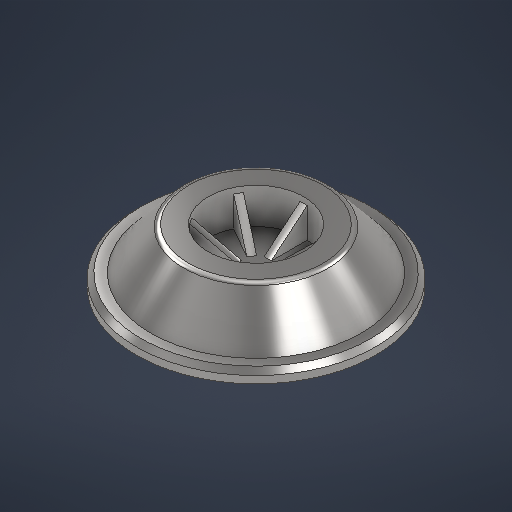
# Autodesk Inventor part: ensayo11
Saved by Autodesk Inventor 2026.2 (Build 302298000, 298)
## iProperties
Created: 2025-12-23
Part Number: ensayo11
Material: Acero inoxidable
Document SubType Name: Modeling
Designer: vicho
Mass: 6174.44 g
Surface Area: 865.841 cm^2
Volume: 771.805 cm^3
Density: 8 g/cm^3
Appearance: Semipulido
Author: vicho
Autodesk Inventor part; units mm, degrees
note: some values were not read from the file. Chosen so that the rebuilt part matches the saved one: direction of "Repujado1".
ref_plane "YZ Plane" through (0, 0, 0) normal (1, 0, 0) x (0, 1, 0)
ref_plane "XY Plane" through (0, 0, 0) normal (0, 0, 1) x (1, 0, 0)
sketch "Boceto1" plane through (0, 0, 0) normal (0, 0, 1) x (1, 0, 0)
  line L0 (0, 50) -> (0, -50) construction
  line L1 (75, 0) -> (-75, 0) construction
  line L2 (-100, 0) -> (-100, 10)
  line L3 (-100, 10) -> (-88, 10)
  line L4 (-88, 10) -> (-58.7804, 45)
  line L5 (-58.7804, 45) -> (-40, 45)
  line L6 (-40, 45) -> (-40, 40.173)
  line L7 (-40, 40.173) -> (-10, 15)
  line L8 (-10, 15) -> (0, 15)
  line L9 (-100, 0) -> (0, 0)
  line L10 (0, 15) -> (-75.8865, 15) construction
  line L11 (0, 15) -> (0, 0)
  dimension "d0" = 150
  dimension "d1" = 100
  dimension "d4" = 10
  dimension "d5" = 15
  dimension "d6" = 10
  dimension "d7" = 12
  dimension "d8" = 45
  dimension "d9" = 40
  dimension "d10" = 40
  dimension "d11" = 100
  dimension "d14" = 39.857
  dimension "d15" = 0
  dimension "d16" = 75.8865
  constraints: 24 end point, 3 perpendicular, 3 point on line, 2 parallel, 2 symmetric about line, 2 vertical, 1 horizontal, 1 midpoint
  measures "d0" distance of L1.start L1.end
  measures "d1" distance of L0.end L0.start
  measures "d4" distance from line of L0 L7.end
  measures "d5" distance between parallel lines of L1 L8
  measures "d6" distance from line of L9 L2.end
  measures "d7" distance of L3.end L2.end
  measures "d8" distance between parallel lines of L1 L5
  measures "d9" distance between parallel lines of L0 L6
  measures "d10" angle of L10 L7
  measures "d11" distance between parallel lines of L0 L2
  measures "d14" angle of L4 L0
  measures "d15" distance from line of L9.end L0
  measures "d16" distance from line of L10.end L0
revolve "Revolución1" add sketch "Boceto1" angle 360 about axis through (0, 50, 0) along (0, -1, 0)
fillet "Empalme1" radius 5 1 edges at (58.7804, 45, 0)
chamfer "Chaflán1" distance 4 angle 45 1 edges at (100, 10, 0)
ref_plane "Plano de trabajo1" through (0, 45, 0) normal (0, 1, 0) x (-1, 0, 0)
sketch "Boceto2" plane through (0, 45, 0) normal (0, 1, 0) x (-1, 0, 0)
  line L0 (0, 63.6119) -> (0, -62.4959) construction
  line L1 (-64.3931, 0) -> (90.5075, 0) construction
  circle A0 centre (0, 0) radius 10 projected
  circle A1 centre (0, 0) radius 40
  line L2 (-3, -39.8873) -> (-3, -9.8873)
  line L3 (-3, -9.8873) -> (3, -9.8873)
  line L4 (3, -9.8873) -> (3, -39.8873)
  line L5 (10.0627, -2.3456) -> (36.0435, -17.3456)
  line L6 (33.0435, -22.5417) -> (7.0627, -7.5417)
  line L7 (7.0627, -7.5417) -> (10.0627, -2.3456)
  circle A2 centre (0, 0) radius 40
  line L8 (7.0627, 7.5417) -> (33.0435, 22.5417)
  line L9 (36.0435, 17.3456) -> (10.0627, 2.3456)
  line L10 (10.0627, 2.3456) -> (7.0627, 7.5417)
  circle A3 centre (0, 0) radius 40
  line L11 (-3, 9.8873) -> (-3, 39.8873)
  line L12 (3, 39.8873) -> (3, 9.8873)
  line L13 (3, 9.8873) -> (-3, 9.8873)
  circle A4 centre (0, 0) radius 40
  line L14 (-10.0627, 2.3456) -> (-36.0435, 17.3456)
  line L15 (-33.0435, 22.5417) -> (-7.0627, 7.5417)
  line L16 (-7.0627, 7.5417) -> (-10.0627, 2.3456)
  circle A5 centre (0, 0) radius 40
  line L17 (-7.0627, -7.5417) -> (-33.0435, -22.5417)
  line L18 (-36.0435, -17.3456) -> (-10.0627, -2.3456)
  line L19 (-10.0627, -2.3456) -> (-7.0627, -7.5417)
  circle A6 centre (0, 0) radius 40
  point P0 (-9.3111, -3.6474)
  point P1 (-9.3111, 3.6474)
  point P2 (-7.8143, -6.24)
  point P3 (-1.4968, -9.8873)
  point P4 (7.8143, -6.24)
  point P5 (1.4968, -9.8873)
  point P6 (9.3111, 3.6474)
  point P7 (9.3111, -3.6474)
  point P8 (-7.8143, 6.24)
  point P9 (-1.4968, 9.8873)
  point P10 (1.4968, 9.8873)
  point P11 (7.8143, 6.24)
  dimension "d23" = 80
  dimension "d24" = 6
  dimension "d25" = 30
  dimension "d28" = 360
  constraints: 40 end point, 12 point on circle, 6 centre point, 2 horizontal, 2 perpendicular, 2 vertical, 1 coincident, 1 parallel, 56 other
  measures "d23" diameter of A1
  measures "d24" distance between parallel lines of L4 L2
  measures "d25" distance from line of L2.start L3
extrude "Extrusión1" cut sketch "Boceto2" against normal blind 30 contours A0 L10 L9 A1 L5 L7 | A0 L13 L12 A1 L8 L10 | L7 L6 A1 L4 L3 A0 | A0 L16 L15 A1 L11 L13 | L3 L2 A1 L17 L19 A0 | A0 L19 L18 A1 L14 L16
sketch "Boceto3" plane through (0, 0, 0) normal (0, -1, 0) x (1, 0, 0)
  line L0 (0.5512, 0) -> (66.3296, 0) construction
  line L1 (66.3296, 0) -> (66.3296, -47.772) construction
  line L2 (66.3296, -47.772) -> (0.5512, -47.772) construction
  line L3 (0.5512, -47.772) -> (0.5512, 0) construction
  line L4 (0.454, -15.6686) -> (5.5107, -0.6686)
  line L5 (5.5107, -0.6686) -> (7.9661, -0.6686)
  line L6 (7.9661, -0.6686) -> (13.0229, -15.6686)
  line L7 (13.0229, -15.6686) -> (10.9199, -15.6686)
  line L8 (10.9199, -15.6686) -> (9.5585, -11.4749)
  line L9 (9.5585, -11.4749) -> (3.8332, -11.4749)
  line L10 (3.8332, -11.4749) -> (2.4718, -15.6686)
  line L11 (2.4718, -15.6686) -> (0.454, -15.6686)
  line L12 (9.0115, -9.7731) -> (6.6898, -2.7107)
  line L13 (6.6898, -2.7107) -> (4.3802, -9.7731)
  line L14 (4.3802, -9.7731) -> (9.0115, -9.7731)
  line L15 (23.0512, -15.6686) -> (21.1549, -15.6686)
  line L16 (21.1549, -15.6686) -> (21.1549, -14.4287)
  spline S0 degree 2 poles (21.1549, -14.4287) (20.2797, -15.1945) (18.7117, -15.9846) (17.7392, -15.9846) knots 0 0 0 1 2 2 2
  spline S1 degree 2 poles (17.7392, -15.9846) (17.0099, -15.9846) (15.7092, -15.4984) (15.2352, -14.9757) knots 0 0 0 1 2 2 2
  spline S2 degree 2 poles (15.2352, -14.9757) (14.7489, -14.453) (14.2141, -12.8606) (14.2141, -11.718) knots 0 0 0 1 2 2 2
  line L17 (14.2141, -11.718) -> (14.2141, -4.4125)
  line L18 (14.2141, -4.4125) -> (16.1104, -4.4125)
  line L19 (16.1104, -4.4125) -> (16.1104, -10.8306)
  spline S3 degree 2 poles (16.1104, -10.8306) (16.1104, -11.7301) (16.2441, -12.9092) (16.475, -13.3468) knots 0 0 0 1 2 2 2
  spline S4 degree 2 poles (16.475, -13.3468) (16.706, -13.7844) (17.4961, -14.1856) (18.2376, -14.1856) knots 0 0 0 1 2 2 2
  spline S5 degree 2 poles (18.2376, -14.1856) (18.9305, -14.1856) (20.4985, -13.3955) (21.1549, -12.8241) knots 0 0 0 1 2 2 2
  line L20 (21.1549, -12.8241) -> (21.1549, -4.4125)
  line L21 (21.1549, -4.4125) -> (23.0512, -4.4125)
  line L22 (23.0512, -4.4125) -> (23.0512, -15.6686)
  spline S6 degree 2 poles (29.2019, -15.8874) (27.6582, -15.8874) (25.9199, -14.1248) (25.9199, -12.2164) knots 0 0 0 1 2 2 2
  line L23 (25.9199, -12.2164) -> (25.9199, -5.9806)
  line L24 (25.9199, -5.9806) -> (24.6436, -5.9806)
  line L25 (24.6436, -5.9806) -> (24.6436, -4.4125)
  line L26 (24.6436, -4.4125) -> (25.9199, -4.4125)
  line L27 (25.9199, -4.4125) -> (25.9199, -1.1791)
  line L28 (25.9199, -1.1791) -> (27.8162, -1.1791)
  line L29 (27.8162, -1.1791) -> (27.8162, -4.4125)
  line L30 (27.8162, -4.4125) -> (31.3049, -4.4125)
  line L31 (31.3049, -4.4125) -> (31.3049, -5.9806)
  line L32 (31.3049, -5.9806) -> (27.8162, -5.9806)
  line L33 (27.8162, -5.9806) -> (27.8162, -11.3412)
  spline S7 degree 2 poles (27.8162, -11.3412) (27.8162, -12.1921) (27.877, -13.128) (28.0836, -13.5292) knots 0 0 0 1 2 2 2
  spline S8 degree 2 poles (28.0836, -13.5292) (28.2538, -13.8817) (29.0196, -14.2342) (29.676, -14.2342) knots 0 0 0 1 2 2 2
  spline S9 degree 2 poles (29.676, -14.2342) (30.1379, -14.2342) (31.001, -13.9546) (31.1955, -13.8695) knots 0 0 0 1 2 2 2
  line L34 (31.1955, -13.8695) -> (31.3049, -13.8695)
  line L35 (31.3049, -13.8695) -> (31.3049, -15.5713)
  spline S10 degree 2 poles (31.3049, -15.5713) (30.77, -15.7172) (29.676, -15.8874) (29.2019, -15.8874) knots 0 0 0 1 2 2 2
  spline S11 degree 2 poles (41.9532, -10.0405) (41.9532, -12.8849) (39.2182, -15.9846) (36.9329, -15.9846) knots 0 0 0 1 2 2 2
  spline S12 degree 2 poles (36.9329, -15.9846) (34.5869, -15.9846) (31.9005, -12.7877) (31.9005, -10.0405) knots 0 0 0 1 2 2 2
  spline S13 degree 2 poles (31.9005, -10.0405) (31.9005, -7.2204) (34.672, -4.0964) (36.9329, -4.0964) knots 0 0 0 1 2 2 2
  spline S14 degree 2 poles (36.9329, -4.0964) (39.2182, -4.0964) (41.9532, -7.2083) (41.9532, -10.0405) knots 0 0 0 1 2 2 2
  spline S15 degree 2 poles (39.9961, -10.0405) (39.9961, -7.8525) (38.4037, -5.7253) (36.9329, -5.7253) knots 0 0 0 1 2 2 2
  spline S16 degree 2 poles (36.9329, -5.7253) (35.4621, -5.7253) (33.8575, -7.8525) (33.8575, -10.0405) knots 0 0 0 1 2 2 2
  spline S17 degree 2 poles (33.8575, -10.0405) (33.8575, -12.1677) (35.4621, -14.3558) (36.9329, -14.3558) knots 0 0 0 1 2 2 2
  spline S18 degree 2 poles (36.9329, -14.3558) (38.3916, -14.3558) (39.9961, -12.2042) (39.9961, -10.0405) knots 0 0 0 1 2 2 2
  line L36 (52.5528, -15.6686) -> (50.6566, -15.6686)
  line L37 (50.6566, -15.6686) -> (50.6566, -14.5259)
  spline S19 degree 2 poles (50.6566, -14.5259) (50.219, -14.8906) (49.5747, -15.3768) (49.1371, -15.5835) knots 0 0 0 1 2 2 2
  spline S20 degree 2 poles (49.1371, -15.5835) (48.736, -15.778) (47.8729, -15.9846) (47.3016, -15.9846) knots 0 0 0 1 2 2 2
  spline S21 degree 2 poles (47.3016, -15.9846) (46.3778, -15.9846) (44.8219, -15.2188) (44.2749, -14.4773) knots 0 0 0 1 2 2 2
  spline S22 degree 2 poles (44.2749, -14.4773) (43.7279, -13.7358) (43.1201, -11.5478) (43.1201, -10.1256) knots 0 0 0 1 2 2 2
  spline S23 degree 2 poles (43.1201, -10.1256) (43.1201, -8.6426) (43.8859, -6.4789) (44.5545, -5.6645) knots 0 0 0 1 2 2 2
  spline S24 degree 2 poles (44.5545, -5.6645) (45.1744, -4.9352) (46.9126, -4.0964) (47.8729, -4.0964) knots 0 0 0 1 2 2 2
  spline S25 degree 2 poles (47.8729, -4.0964) (48.7117, -4.0964) (49.9637, -4.4733) (50.6566, -4.8622) knots 0 0 0 1 2 2 2
  line L38 (50.6566, -4.8622) -> (50.6566, 0)
  line L39 (50.6566, 0) -> (52.5528, 0)
  line L40 (52.5528, 0) -> (52.5528, -15.6686)
  line L41 (50.6566, -12.9335) -> (50.6566, -6.4303)
  spline S26 degree 2 poles (50.6566, -6.4303) (49.9515, -6.09) (48.8332, -5.8347) (48.189, -5.8347) knots 0 0 0 1 2 2 2
  spline S27 degree 2 poles (48.189, -5.8347) (46.7303, -5.8347) (45.0771, -8.0227) (45.0771, -10.0891) knots 0 0 0 1 2 2 2
  spline S28 degree 2 poles (45.0771, -10.0891) (45.0771, -12.0827) (46.3413, -14.1856) (47.7392, -14.1856) knots 0 0 0 1 2 2 2
  spline S29 degree 2 poles (47.7392, -14.1856) (48.4807, -14.1856) (49.988, -13.5049) (50.6566, -12.9335) knots 0 0 0 1 2 2 2
  spline S30 degree 2 poles (60.1865, -15.9238) (57.488, -15.9238) (54.522, -12.8971) (54.522, -10.1013) knots 0 0 0 1 2 2 2
  spline S31 degree 2 poles (54.522, -10.1013) (54.522, -7.3541) (57.4029, -4.0964) (59.7246, -4.0964) knots 0 0 0 1 2 2 2
  spline S32 degree 2 poles (59.7246, -4.0964) (60.77, -4.0964) (62.3867, -4.7042) (62.9823, -5.3485) knots 0 0 0 1 2 2 2
  spline S33 degree 2 poles (62.9823, -5.3485) (63.5901, -5.9927) (64.2344, -7.8525) (64.2344, -9.2018) knots 0 0 0 1 2 2 2
  line L42 (64.2344, -9.2018) -> (64.2344, -10.235)
  line L43 (64.2344, -10.235) -> (56.4426, -10.235)
  spline S34 degree 2 poles (56.4426, -10.235) (56.4426, -12.1921) (58.4118, -14.2707) (60.1622, -14.2707) knots 0 0 0 1 2 2 2
  spline S35 degree 2 poles (60.1622, -14.2707) (60.7822, -14.2707) (61.9856, -13.9911) (62.4718, -13.7723) knots 0 0 0 1 2 2 2
  spline S36 degree 2 poles (62.4718, -13.7723) (62.9823, -13.5292) (63.6874, -13.1037) (63.9183, -12.9092) knots 0 0 0 1 2 2 2
  line L44 (63.9183, -12.9092) -> (64.0277, -12.9092)
  line L45 (64.0277, -12.9092) -> (64.0277, -14.9757)
  spline S37 degree 2 poles (64.0277, -14.9757) (63.6995, -15.1094) (62.7028, -15.4984) (62.3138, -15.6078) knots 0 0 0 1 2 2 2
  spline S38 degree 2 poles (62.3138, -15.6078) (61.7668, -15.7658) (60.8673, -15.9238) (60.1865, -15.9238) knots 0 0 0 1 2 2 2
  spline S39 degree 2 poles (62.3867, -8.7885) (62.3624, -8.0227) (62.0464, -6.9044) (61.7425, -6.5276) knots 0 0 0 1 2 2 2
  spline S40 degree 2 poles (61.7425, -6.5276) (61.4143, -6.1021) (60.381, -5.6524) (59.6152, -5.6524) knots 0 0 0 1 2 2 2
  spline S41 degree 2 poles (59.6152, -5.6524) (58.8616, -5.6524) (57.8041, -6.1021) (57.3665, -6.5397) knots 0 0 0 1 2 2 2
  spline S42 degree 2 poles (57.3665, -6.5397) (56.941, -6.9895) (56.5034, -8.0713) (56.4426, -8.7885) knots 0 0 0 1 2 2 2
  line L46 (56.4426, -8.7885) -> (62.3867, -8.7885)
  spline S43 degree 2 poles (69.1938, -15.936) (68.0634, -15.936) (66.1063, -15.3282) (65.4621, -14.9878) knots 0 0 0 1 2 2 2
  line L47 (65.4621, -14.9878) -> (65.4621, -12.8606)
  line L48 (65.4621, -12.8606) -> (65.5593, -12.8606)
  spline S44 degree 2 poles (65.5593, -12.8606) (65.8024, -13.0551) (66.4588, -13.517) (67.0058, -13.7723) knots 0 0 0 1 2 2 2
  spline S45 degree 2 poles (67.0058, -13.7723) (67.4799, -14.0032) (68.6468, -14.3436) (69.2668, -14.3436) knots 0 0 0 1 2 2 2
  spline S46 degree 2 poles (69.2668, -14.3436) (69.7165, -14.3436) (70.7498, -14.137) (70.9929, -13.9668) knots 0 0 0 1 2 2 2
  spline S47 degree 2 poles (70.9929, -13.9668) (71.3454, -13.7358) (71.6614, -13.2131) (71.6614, -12.6783) knots 0 0 0 1 2 2 2
  spline S48 degree 2 poles (71.6614, -12.6783) (71.6614, -12.0097) (70.9321, -11.3169) (69.9961, -11.0859) knots 0 0 0 1 2 2 2
  spline S49 degree 2 poles (69.9961, -11.0859) (69.6314, -11.0008) (68.4645, -10.7577) (67.9661, -10.624) knots 0 0 0 1 2 2 2
  spline S50 degree 2 poles (67.9661, -10.624) (66.6776, -10.2472) (65.5107, -8.6912) (65.5107, -7.5851) knots 0 0 0 1 2 2 2
  spline S51 degree 2 poles (65.5107, -7.5851) (65.5107, -6.0535) (67.8081, -4.1451) (69.7044, -4.1451) knots 0 0 0 1 2 2 2
  spline S52 degree 2 poles (69.7044, -4.1451) (70.6404, -4.1451) (72.5366, -4.607) (73.1809, -4.9595) knots 0 0 0 1 2 2 2
  line L49 (73.1809, -4.9595) -> (73.1809, -6.9895)
  line L50 (73.1809, -6.9895) -> (73.0836, -6.9895)
  spline S53 degree 2 poles (73.0836, -6.9895) (72.3543, -6.406) (70.5796, -5.7374) (69.6679, -5.7374) knots 0 0 0 1 2 2 2
  spline S54 degree 2 poles (69.6679, -5.7374) (68.7319, -5.7374) (67.4434, -6.5276) (67.4434, -7.3177) knots 0 0 0 1 2 2 2
  spline S55 degree 2 poles (67.4434, -7.3177) (67.4434, -8.0348) (68.2092, -8.7277) (69.0601, -8.9465) knots 0 0 0 1 2 2 2
  spline S56 degree 2 poles (69.0601, -8.9465) (69.4734, -9.0559) (70.5188, -9.2747) (71.0901, -9.4084) knots 0 0 0 1 2 2 2
  spline S57 degree 2 poles (71.0901, -9.4084) (72.33, -9.7245) (73.5942, -11.171) (73.5942, -12.423) knots 0 0 0 1 2 2 2
  spline S58 degree 2 poles (73.5942, -12.423) (73.5942, -13.1524) (73.0229, -14.4408) (72.4637, -14.9149) knots 0 0 0 1 2 2 2
  spline S59 degree 2 poles (72.4637, -14.9149) (71.8681, -15.4133) (70.3486, -15.936) (69.1938, -15.936) knots 0 0 0 1 2 2 2
  line L51 (84.6801, -15.6686) -> (82.1882, -15.6686)
  line L52 (82.1882, -15.6686) -> (78.0066, -10.235)
  line L53 (78.0066, -10.235) -> (77.253, -10.9643)
  line L54 (77.253, -10.9643) -> (77.253, -15.6686)
  line L55 (77.253, -15.6686) -> (75.3567, -15.6686)
  line L56 (75.3567, -15.6686) -> (75.3567, 0)
  line L57 (75.3567, 0) -> (77.253, 0)
  line L58 (77.253, 0) -> (77.253, -9.1653)
  line L59 (77.253, -9.1653) -> (81.7019, -4.4125)
  line L60 (81.7019, -4.4125) -> (84.0601, -4.4125)
  line L61 (84.0601, -4.4125) -> (79.441, -9.1167)
  line L62 (79.441, -9.1167) -> (84.6801, -15.6686)
  line L63 (7.2976, -40.3657) -> (1.4872, -40.3657)
  line L64 (1.4872, -40.3657) -> (1.4872, -38.8341)
  line L65 (1.4872, -38.8341) -> (3.3956, -38.8341)
  line L66 (3.3956, -38.8341) -> (3.3956, -26.8973)
  line L67 (3.3956, -26.8973) -> (1.4872, -26.8973)
  line L68 (1.4872, -26.8973) -> (1.4872, -25.3657)
  line L69 (1.4872, -25.3657) -> (7.2976, -25.3657)
  line L70 (7.2976, -25.3657) -> (7.2976, -26.8973)
  line L71 (7.2976, -26.8973) -> (5.3891, -26.8973)
  line L72 (5.3891, -26.8973) -> (5.3891, -38.8341)
  line L73 (5.3891, -38.8341) -> (7.2976, -38.8341)
  line L74 (7.2976, -38.8341) -> (7.2976, -40.3657)
  line L75 (18.4564, -40.3657) -> (16.5601, -40.3657)
  line L76 (16.5601, -40.3657) -> (16.5601, -33.9475)
  spline S60 degree 2 poles (16.5601, -33.9475) (16.5601, -33.1696) (16.4143, -31.8324) (16.1955, -31.4313) knots 0 0 0 1 2 2 2
  spline S61 degree 2 poles (16.1955, -31.4313) (15.9645, -31.0059) (15.1379, -30.5926) (14.4329, -30.5926) knots 0 0 0 1 2 2 2
  spline S62 degree 2 poles (14.4329, -30.5926) (13.7279, -30.5926) (12.2327, -31.3462) (11.5156, -31.954) knots 0 0 0 1 2 2 2
  line L77 (11.5156, -31.954) -> (11.5156, -40.3657)
  line L78 (11.5156, -40.3657) -> (9.6193, -40.3657)
  line L79 (9.6193, -40.3657) -> (9.6193, -29.1096)
  line L80 (9.6193, -29.1096) -> (11.5156, -29.1096)
  line L81 (11.5156, -29.1096) -> (11.5156, -30.3616)
  spline S63 degree 2 poles (11.5156, -30.3616) (12.3665, -29.5958) (14.0075, -28.7935) (14.9313, -28.7935) knots 0 0 0 1 2 2 2
  spline S64 degree 2 poles (14.9313, -28.7935) (16.5844, -28.7935) (18.4564, -30.9815) (18.4564, -33.0602) knots 0 0 0 1 2 2 2
  line L82 (18.4564, -33.0602) -> (18.4564, -40.3657)
  line L83 (29.9556, -29.1096) -> (25.7133, -40.3657)
  line L84 (25.7133, -40.3657) -> (24.0115, -40.3657)
  line L85 (24.0115, -40.3657) -> (19.8057, -29.1096)
  line L86 (19.8057, -29.1096) -> (21.86, -29.1096)
  line L87 (21.86, -29.1096) -> (24.9353, -37.7765)
  line L88 (24.9353, -37.7765) -> (27.9864, -29.1096)
  line L89 (27.9864, -29.1096) -> (29.9556, -29.1096)
  spline S65 degree 2 poles (36.2765, -40.6209) (33.578, -40.6209) (30.612, -37.5942) (30.612, -34.7984) knots 0 0 0 1 2 2 2
  spline S66 degree 2 poles (30.612, -34.7984) (30.612, -32.0512) (33.4929, -28.7935) (35.8146, -28.7935) knots 0 0 0 1 2 2 2
  spline S67 degree 2 poles (35.8146, -28.7935) (36.86, -28.7935) (38.4767, -29.4013) (39.0723, -30.0456) knots 0 0 0 1 2 2 2
  spline S68 degree 2 poles (39.0723, -30.0456) (39.6801, -30.6898) (40.3243, -32.5496) (40.3243, -33.8989) knots 0 0 0 1 2 2 2
  line L90 (40.3243, -33.8989) -> (40.3243, -34.9321)
  line L91 (40.3243, -34.9321) -> (32.5326, -34.9321)
  spline S69 degree 2 poles (32.5326, -34.9321) (32.5326, -36.8892) (34.5018, -38.9678) (36.2522, -38.9678) knots 0 0 0 1 2 2 2
  spline S70 degree 2 poles (36.2522, -38.9678) (36.8721, -38.9678) (38.0755, -38.6882) (38.5618, -38.4694) knots 0 0 0 1 2 2 2
  spline S71 degree 2 poles (38.5618, -38.4694) (39.0723, -38.2263) (39.7773, -37.8008) (40.0083, -37.6063) knots 0 0 0 1 2 2 2
  line L92 (40.0083, -37.6063) -> (40.1177, -37.6063)
  line L93 (40.1177, -37.6063) -> (40.1177, -39.6728)
  spline S72 degree 2 poles (40.1177, -39.6728) (39.7895, -39.8065) (38.7927, -40.1955) (38.4037, -40.3049) knots 0 0 0 1 2 2 2
  spline S73 degree 2 poles (38.4037, -40.3049) (37.8567, -40.4629) (36.9572, -40.6209) (36.2765, -40.6209) knots 0 0 0 1 2 2 2
  spline S74 degree 2 poles (38.4767, -33.4856) (38.4524, -32.7198) (38.1363, -31.6015) (37.8324, -31.2247) knots 0 0 0 1 2 2 2
  spline S75 degree 2 poles (37.8324, -31.2247) (37.5042, -30.7992) (36.471, -30.3495) (35.7052, -30.3495) knots 0 0 0 1 2 2 2
  spline S76 degree 2 poles (35.7052, -30.3495) (34.9515, -30.3495) (33.894, -30.7992) (33.4564, -31.2368) knots 0 0 0 1 2 2 2
  spline S77 degree 2 poles (33.4564, -31.2368) (33.031, -31.6866) (32.5934, -32.7684) (32.5326, -33.4856) knots 0 0 0 1 2 2 2
  line L94 (32.5326, -33.4856) -> (38.4767, -33.4856)
  line L95 (51.082, -40.3657) -> (49.1857, -40.3657)
  line L96 (49.1857, -40.3657) -> (49.1857, -33.9475)
  spline S78 degree 2 poles (49.1857, -33.9475) (49.1857, -33.1696) (49.0399, -31.8324) (48.8211, -31.4313) knots 0 0 0 1 2 2 2
  spline S79 degree 2 poles (48.8211, -31.4313) (48.5901, -31.0059) (47.7635, -30.5926) (47.0585, -30.5926) knots 0 0 0 1 2 2 2
  spline S80 degree 2 poles (47.0585, -30.5926) (46.3535, -30.5926) (44.8583, -31.3462) (44.1412, -31.954) knots 0 0 0 1 2 2 2
  line L97 (44.1412, -31.954) -> (44.1412, -40.3657)
  line L98 (44.1412, -40.3657) -> (42.2449, -40.3657)
  line L99 (42.2449, -40.3657) -> (42.2449, -29.1096)
  line L100 (42.2449, -29.1096) -> (44.1412, -29.1096)
  line L101 (44.1412, -29.1096) -> (44.1412, -30.3616)
  spline S81 degree 2 poles (44.1412, -30.3616) (44.9921, -29.5958) (46.6331, -28.7935) (47.5569, -28.7935) knots 0 0 0 1 2 2 2
  spline S82 degree 2 poles (47.5569, -28.7935) (49.21, -28.7935) (51.082, -30.9815) (51.082, -33.0602) knots 0 0 0 1 2 2 2
  line L102 (51.082, -33.0602) -> (51.082, -40.3657)
  spline S83 degree 2 poles (57.1477, -40.5845) (55.6039, -40.5845) (53.8656, -38.8219) (53.8656, -36.9135) knots 0 0 0 1 2 2 2
  line L103 (53.8656, -36.9135) -> (53.8656, -30.6777)
  line L104 (53.8656, -30.6777) -> (52.5893, -30.6777)
  line L105 (52.5893, -30.6777) -> (52.5893, -29.1096)
  line L106 (52.5893, -29.1096) -> (53.8656, -29.1096)
  line L107 (53.8656, -29.1096) -> (53.8656, -25.8762)
  line L108 (53.8656, -25.8762) -> (55.7619, -25.8762)
  line L109 (55.7619, -25.8762) -> (55.7619, -29.1096)
  line L110 (55.7619, -29.1096) -> (59.2506, -29.1096)
  line L111 (59.2506, -29.1096) -> (59.2506, -30.6777)
  line L112 (59.2506, -30.6777) -> (55.7619, -30.6777)
  line L113 (55.7619, -30.6777) -> (55.7619, -36.0383)
  spline S84 degree 2 poles (55.7619, -36.0383) (55.7619, -36.8892) (55.8227, -37.8251) (56.0293, -38.2263) knots 0 0 0 1 2 2 2
  spline S85 degree 2 poles (56.0293, -38.2263) (56.1995, -38.5788) (56.9653, -38.9313) (57.6217, -38.9313) knots 0 0 0 1 2 2 2
  spline S86 degree 2 poles (57.6217, -38.9313) (58.0836, -38.9313) (58.9467, -38.6517) (59.1412, -38.5666) knots 0 0 0 1 2 2 2
  line L114 (59.1412, -38.5666) -> (59.2506, -38.5666)
  line L115 (59.2506, -38.5666) -> (59.2506, -40.2684)
  spline S87 degree 2 poles (59.2506, -40.2684) (58.7157, -40.4143) (57.6217, -40.5845) (57.1477, -40.5845) knots 0 0 0 1 2 2 2
  spline S88 degree 2 poles (69.8989, -34.7376) (69.8989, -37.582) (67.1639, -40.6817) (64.8786, -40.6817) knots 0 0 0 1 2 2 2
  spline S89 degree 2 poles (64.8786, -40.6817) (62.5326, -40.6817) (59.8462, -37.4848) (59.8462, -34.7376) knots 0 0 0 1 2 2 2
  spline S90 degree 2 poles (59.8462, -34.7376) (59.8462, -31.9175) (62.6177, -28.7935) (64.8786, -28.7935) knots 0 0 0 1 2 2 2
  spline S91 degree 2 poles (64.8786, -28.7935) (67.1639, -28.7935) (69.8989, -31.9054) (69.8989, -34.7376) knots 0 0 0 1 2 2 2
  spline S92 degree 2 poles (67.9418, -34.7376) (67.9418, -32.5496) (66.3494, -30.4224) (64.8786, -30.4224) knots 0 0 0 1 2 2 2
  spline S93 degree 2 poles (64.8786, -30.4224) (63.4078, -30.4224) (61.8032, -32.5496) (61.8032, -34.7376) knots 0 0 0 1 2 2 2
  spline S94 degree 2 poles (61.8032, -34.7376) (61.8032, -36.8649) (63.4078, -39.0529) (64.8786, -39.0529) knots 0 0 0 1 2 2 2
  spline S95 degree 2 poles (64.8786, -39.0529) (66.3373, -39.0529) (67.9418, -36.9013) (67.9418, -34.7376) knots 0 0 0 1 2 2 2
  line L116 (77.8122, -31.1396) -> (77.7149, -31.1396)
  spline S96 degree 2 poles (77.7149, -31.1396) (77.4961, -31.0788) (77.022, -31.0545) (76.6938, -31.0545) knots 0 0 0 1 2 2 2
  spline S97 degree 2 poles (76.6938, -31.0545) (75.928, -31.0545) (74.4207, -31.723) (73.74, -32.3794) knots 0 0 0 1 2 2 2
  line L117 (73.74, -32.3794) -> (73.74, -40.3657)
  line L118 (73.74, -40.3657) -> (71.8438, -40.3657)
  line L119 (71.8438, -40.3657) -> (71.8438, -29.1096)
  line L120 (71.8438, -29.1096) -> (73.74, -29.1096)
  line L121 (73.74, -29.1096) -> (73.74, -30.7871)
  spline S98 degree 2 poles (73.74, -30.7871) (74.7733, -29.8632) (76.317, -29.1096) (77.0464, -29.1096) knots 0 0 0 1 2 2 2
  spline S99 degree 2 poles (77.0464, -29.1096) (77.3381, -29.1096) (77.6298, -29.1339) (77.8122, -29.1704) knots 0 0 0 1 2 2 2
  line L122 (77.8122, -29.1704) -> (77.8122, -31.1396)
  point P0 (0, 0)
  constraints: 2 other
emboss "Repujado1" sketch "Boceto3" operation add depth 1 direction (0, 1, 0)
